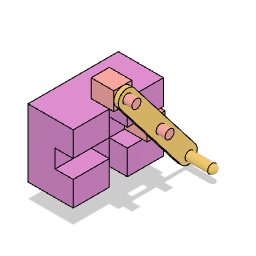
Suma 2004 v1 (Autodesk Fusion 360 design; units mm, degrees)
Autodesk Fusion 360 part; units mm, degrees
sketch "Sketch1" plane through (0, 0, 0) normal (1, 0, 0) x (0, 0, -1)
  line L0 (0, 0) -> (200, 0)
  line L1 (200, 0) -> (200, -150)
  line L2 (200, -150) -> (0, -150)
  line L3 (0, -150) -> (0, 0)
  dimension "d1" = 200
  dimension "d2" = 150
  constraint horizontal L0
  constraint vertical L1
  constraint horizontal L2
  constraint vertical L3
  constraint coincident L0.start L3.end
  measures "d1" distance of L0.start L0.end
  measures "d2" distance of L0.start L2.end
extrude "Extrude1" add sketch "Sketch1" along normal blind 100 makes body 1
sketch "Sketch2" plane through (100, 0, 0) normal (1, 0, 0) x (0, 0, -1)
  line L0 (0, -150) -> (200, -150)
  line L1 (200, -150) -> (200, 0)
  line L2 (200, 0) -> (0, 0)
  line L3 (0, 0) -> (0, -150)
  line L4 (100, -20) -> (100, -140)
  line L5 (20, -75) -> (170, -75)
  line L6 (80, 30) -> (120, 30)
  line L7 (120, 30) -> (120, -175.2632)
  line L8 (120, -175.2632) -> (80, -175.2632)
  line L9 (80, -175.2632) -> (80, 30)
  line L10 (-30, -55) -> (232.2693, -55)
  line L11 (232.2693, -55) -> (232.2693, -95)
  line L12 (232.2693, -95) -> (-30, -95)
  line L13 (-30, -95) -> (-30, -55)
  dimension "d5" = 40
  dimension "d6" = 40
  constraint vertical L4
  constraint horizontal L5
  constraint symmetric L0 L2 L5
  constraint symmetric L1 L3 L4
  constraint horizontal L6
  constraint vertical L7
  constraint horizontal L8
  constraint vertical L9
  constraint horizontal L10
  constraint vertical L11
  constraint horizontal L12
  constraint vertical L13
  constraint symmetric L4 L7 L9
  constraint symmetric L5 L10 L12
  measures "d5" distance of L6.start L6.end
  measures "d6" distance of L10.end L11.end
extrude "Extrude2" cut sketch "Sketch2" against normal blind 40 contours L0 L7 L9 L12 | L3 L9 L10 L12 | L4 L5 L9 L12 | L4 L5 L7 L12 | L1 L7 L10 L12 | L4 L5 L9 L10 | L2 L7 L9 L10 | L4 L5 L7 L10 bodies 1
sketch "Sketch3" plane through (60, 0, 0) normal (1, 0, 0) x (0, 0, -1)
  line L0 (120, -95) -> (200, -95)
  line L1 (200, -95) -> (200, -55)
  line L2 (200, -55) -> (120, -55)
  line L3 (120, -55) -> (120, 0)
  line L4 (120, 0) -> (80, 0)
  line L5 (80, 0) -> (80, -55)
  line L6 (80, -55) -> (0, -55)
  line L7 (0, -55) -> (0, -95)
  line L8 (0, -95) -> (80, -95)
  line L9 (80, -95) -> (80, -150)
  line L10 (80, -150) -> (120, -150)
  line L11 (120, -150) -> (120, -95)
  line L12 (80, 0) -> (120, 0)
  line L13 (120, 0) -> (120, -40)
  line L14 (120, -40) -> (80, -40)
  line L15 (80, -40) -> (80, 0)
  line L16 (200, -55) -> (160, -55)
  line L17 (160, -55) -> (160, -95)
  line L18 (160, -95) -> (200, -95)
  line L19 (200, -95) -> (200, -55)
  line L20 (80, -150) -> (120, -150)
  line L21 (120, -150) -> (120, -110)
  line L22 (120, -110) -> (80, -110)
  line L23 (80, -110) -> (80, -150)
  line L24 (0, -55) -> (40, -55)
  line L25 (40, -55) -> (40, -95)
  line L26 (40, -95) -> (0, -95)
  line L27 (0, -95) -> (0, -55)
  dimension "d9" = 40
  dimension "d10" = 40
  constraint horizontal L12
  constraint vertical L13
  constraint horizontal L14
  constraint vertical L15
  constraint coincident L3 L13.end
  constraint coincident L4.end L5.start
  constraint horizontal L16
  constraint vertical L17
  constraint horizontal L18
  constraint vertical L19
  constraint midpoint L0 L17.end
  constraint coincident L1.end L2.start
  constraint horizontal L20
  constraint vertical L21
  constraint horizontal L22
  constraint vertical L23
  constraint coincident L9.end L10.start
  constraint horizontal L24
  constraint vertical L25
  constraint horizontal L26
  constraint vertical L27
  constraint coincident L6.end L7.start
  measures "d9" distance of L9.end L22.end
  measures "d10" distance of L6.end L24.end
extrude "Extrude1'" add sketch "Sketch3" along normal blind 50 separate body contours L0 L1 L2 L16 L17 L18 L19 makes body 2 in component "Component"
sketch "Sketch4" plane through (110, 0, 0) normal (1, 0, 0) x (0, 0, -1)
  line L0 (200, -95) -> (200, -55)
  line L1 (200, -55) -> (160, -55)
  line L2 (160, -55) -> (160, -95)
  line L3 (160, -95) -> (200, -95)
  circle A0 centre (180, -75) radius 10
  dimension "d13" = 20
  measures "d13" diameter of A0
extrude "Extrude2'" add sketch "Sketch4" along normal blind 30 contours A0 bodies 2 in component "Component"
sketch "Sketch5" plane through (100, 0, 0) normal (1, 0, 0) x (0, 0, -1)
  line L0 (120, 0) -> (120, -55)
  line L1 (120, -55) -> (200, -55)
  line L2 (200, -55) -> (200, 0)
  line L3 (200, 0) -> (120, 0)
  line L4 (70, 50) -> (190, 50)
  line L5 (190, 90) -> (70, 90)
  arc A0 (70, 90) -> (70, 50) centre (70, 70) ccw
  line L6 (70, 70) -> (190, 70) construction
  line L7 (190, 90) -> (310, 90)
  line L8 (310, 90) -> (310, 50)
  line L9 (310, 50) -> (190, 50)
  circle A1 centre (70, 70) radius 10
  circle A2 centre (190, 70) radius 10
  dimension "d16" = 120
  dimension "d18" = 20
  dimension "d19" = 20
  constraint parallel L4 L5
  constraint tangent L5 A0
  constraint tangent L4 A0
  constraint horizontal L6
  constraint perpendicular L4 L8
  constraint concentric A0 A1
  constraint coincident L6.end A2.centre
  measures "d16" distance of A0.centre L6.end
  measures "d18" diameter of A1
  measures "d19" diameter of A2
extrude "Extrude1''" add sketch "Sketch5" along normal blind 10 separate body contours L4 L5 A0 L7 L8 L9 makes body 3 in component "Component'"
sketch "Sketch6" plane through (110, 0, 0) normal (1, 0, 0) x (0, 0, -1)
  circle A0 centre (70, 70) radius 10
  circle A1 centre (190, 70) radius 10
  line L0 (310, 90) -> (70, 90)
  arc A2 (70, 90) -> (70, 50) centre (70, 70) ccw
  line L1 (70, 50) -> (310, 50)
  line L2 (310, 50) -> (310, 90)
  circle A3 centre (295, 70) radius 10
  dimension "d22" = 20
  measures "d22" diameter of A3
extrude "Extrude2''" add sketch "Sketch6" along normal blind 60 contours A3 bodies 3 in component "Component'"
fillet "Fillet1" radius 10 1 edges at (170, 66.3838, -285.6767) on bodies 3 in component "Component'"
fillet "Fillet2" radius 20 2 edges at (105, 50, -310) (105, 90, -310) on bodies 3 in component "Component'"
component "Component" placed x (1, 0, 0) y (0, 1, 0) z (0, 0, 1) at (0, 0, -40)
component "Component" placed x (1, 0, 0) y (0, 1, 0) z (0, 0, 1) at (0, 0, 80)
component "Component'" placed x (1, 0, 0) y (0, 1, 0) z (0, 0, 1) at (10, -145, -30)
